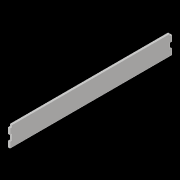
# Autodesk Inventor part: Front V3
Saved by Autodesk Inventor 2018 (Build 220112000, 112)
## iProperties
Created: 2017-09-14
Part Number: Front V3
Material: Generic
Document SubType Name: Modeling
Designer: gaine
Density: 1 g/cm^3
Appearance: Default
Author: gaine
Autodesk Inventor part; units mm, degrees
ref_plane "YZ Plane" through (0, 0, 0) normal (1, 0, 0) x (0, 1, 0)
ref_plane "XZ Plane" through (0, 0, 0) normal (0, 1, 0) x (-1, 0, 0)
ref_plane "XY Plane" through (0, 0, 0) normal (0, 0, 1) x (1, 0, 0)
sketch "Sketch1" plane through (0, 0, 0) normal (1, 0, 0) x (0, 1, 0)
  line L0 (-19.05, 441.8979) -> (-19.05, -99.1221)
  line L1 (45.3898, -92.7721) -> (45.3898, 435.5479)
  line L2 (19.9898, 441.8979) -> (19.9898, 435.5479)
  line L3 (19.9898, 435.5479) -> (0, 435.5479)
  line L4 (0, 435.5479) -> (0, 441.8979)
  line L5 (39.0398, 441.8979) -> (39.0398, 435.5479)
  line L6 (39.0398, 435.5479) -> (45.3898, 435.5479)
  line L7 (39.0398, -99.1221) -> (39.0398, -92.7721)
  line L8 (39.0398, -92.7721) -> (45.3898, -92.7721)
  line L9 (0, -99.1221) -> (0, -92.7721)
  line L10 (0, -92.7721) -> (19.9898, -92.7721)
  line L11 (19.9898, -92.7721) -> (19.9898, -99.1221)
  line L12 (39.0398, 441.8979) -> (19.9898, 441.8979)
  line L13 (0, 441.8979) -> (-19.05, 441.8979)
  line L14 (-19.05, -99.1221) -> (0, -99.1221)
  line L15 (19.9898, -99.1221) -> (39.0398, -99.1221)
  point P0 (0, 0)
  dimension "d12" = 6.35
  dimension "d13" = 6.35
  dimension "d14" = 19.05
  dimension "d15" = 19.9898
  dimension "d16" = 6.35
  dimension "d17" = 64.4398
  dimension "d18" = 6.35
  dimension "d19" = 6.35
  dimension "d20" = 19.05
  dimension "d21" = 19.9898
  dimension "d22" = 6.35
  dimension "d23" = 541.02
  dimension "d26" = 6.35
  constraints: 32 end point, 7 parallel, 2 horizontal, 2 perpendicular
  measures "d12" distance between parallel lines of L15 L8
  measures "d13" distance between parallel lines of L14 L10
  measures "d14" distance between parallel lines of L11 L7
  measures "d15" distance between parallel lines of L9 L11
  measures "d16" distance between parallel lines of L7 L1
  measures "d17" distance between parallel lines of L0 L1
  measures "d18" distance between parallel lines of L12 L6
  measures "d19" distance between parallel lines of L13 L3
  measures "d20" distance between parallel lines of L2 L5
  measures "d21" distance between parallel lines of L4 L2
  measures "d22" distance between parallel lines of L1 L5
  measures "d23" distance between parallel lines of L14 L13
  measures "d26" distance between parallel lines of L12 L3
extrude "Extrusion1" add sketch "Sketch1" along normal blind 6.35
body "Solid1"
